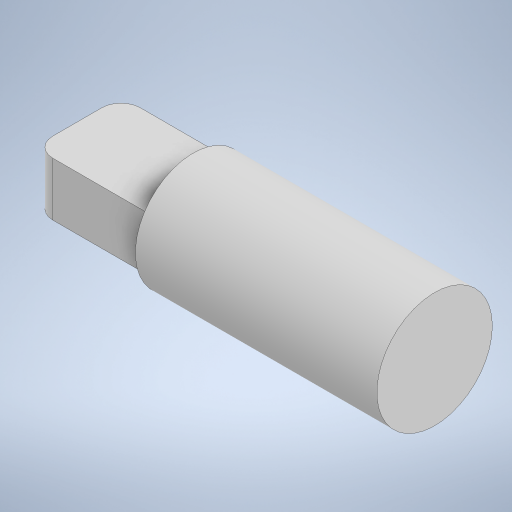
# Autodesk Inventor part: Part6 x 2
Saved by Autodesk Inventor 2023.1 (Build 271208000, 208)
## iProperties
Created: 2022-10-25
Part Number: Part6 x 2
Material: Generic
Document SubType Name: Modeling
Designer: jshin23
Density: 1 g/cm^3
Appearance: Default
Author: jshin23
Autodesk Inventor part; units mm, degrees
ref_plane "YZ Plane" through (0, 0, 0) normal (1, 0, 0) x (0, 1, 0)
ref_plane "XZ Plane" through (0, 0, 0) normal (0, 1, 0) x (-1, 0, 0)
ref_plane "XY Plane" through (0, 0, 0) normal (0, 0, 1) x (1, 0, 0)
sketch "Sketch1" plane through (0, 0, 0) normal (0, 1, 0) x (-1, 0, 0)
  line L0 (0, 0) -> (19.177, 0)
  line L1 (19.177, 0) -> (19.177, -14.478)
  line L2 (19.177, -14.478) -> (0, -14.478)
  line L3 (0, -14.478) -> (0, 0)
  dimension "d0" = 19.177
  dimension "d1" = 14.478
  constraints: 8 end point, 2 parallel, 1 horizontal, 1 perpendicular
  measures "d0" distance of L1.end L2.end
  measures "d1" distance of L0.end L1.end
extrude "Extrusion1" add sketch "Sketch1" along normal blind 8.89
sketch "Sketch2" plane through (0, 0, 0) normal (1, 0, 0) x (0, 0, -1)
  circle A0 centre (7.239, 4.445) radius 9.5631
  line L0 (0, 8.89) -> (14.478, 8.89) projected
  line L1 (0, 0) -> (0, 8.89) projected
  line L2 (14.478, 0) -> (0, 0) projected
  line L3 (0, 0) -> (0, 8.89) projected
  point P0 (7.239, 0)
  point P1 (0, 4.445)
  dimension "d4" = 19.1262
  dimension "d9" = 0
  dimension "d10" = 0
  constraints: 2 midpoint, 1 centre point
  measures "d4" diameter of A0
  measures "d9" horizontal distance of A0.centre point (7.239, 0)
  measures "d10" vertical distance of A0.centre point (0, 4.445)
extrude "Extrusion2" add sketch "Sketch2" along normal blind 40.005
fillet "Fillet1" radius 3.175 2 edges at (-19.177, 4.445, 0) (-19.177, 4.445, -14.478)
body "Solid1"
